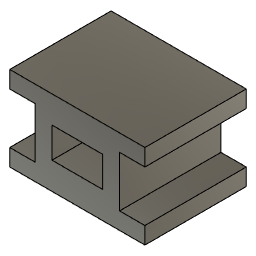
Part 8 (Autodesk Fusion 360 design; units mm, degrees)
Autodesk Fusion 360 part; units mm, degrees
sketch "Sketch2" plane through (0, 0, 0) normal (0, 1, 0) x (1, 0, 0)
  line L0 (40, -25) -> (-40, -25)
  line L1 (-40, -25) -> (-40, 25)
  line L2 (-40, 25) -> (40, 25)
  line L3 (40, 25) -> (40, -25)
  line L4 (40, -25) -> (-40, 25) construction
  line L5 (-40, -25) -> (40, 25) construction
  line L6 (15, -9) -> (-15, -9)
  line L7 (-15, -9) -> (-15, 9)
  line L8 (-15, 9) -> (15, 9)
  line L9 (15, 9) -> (15, -9)
  line L10 (15, -9) -> (-15, 9) construction
  line L11 (-15, -9) -> (15, 9) construction
  line L12 (40, -15) -> (25, -15)
  line L13 (25, -15) -> (25, 15)
  line L14 (25, 15) -> (40, 15)
  line L15 (40, 15) -> (40, -15)
  line L16 (-40, 15) -> (-25, 15)
  line L17 (-25, 15) -> (-25, -15)
  line L18 (-25, -15) -> (-40, -15)
  line L19 (-40, -15) -> (-40, 15)
  dimension "d13" = 80
  dimension "d14" = 50
  dimension "d15" = 30
  dimension "d16" = 18
  dimension "d17" = 15
  dimension "d18" = 30
  dimension "d19" = 10
  constraint horizontal L0
  constraint perpendicular L0 L1
  constraint parallel L0 L2
  constraint parallel L1 L3
  constraint coincident L4 origin
  constraint coincident L5 origin
  constraint horizontal L6
  constraint perpendicular L6 L7
  constraint parallel L6 L8
  constraint parallel L7 L9
  constraint coincident L10 origin
  constraint coincident L11 origin
  constraint horizontal L12
  constraint vertical L13
  constraint horizontal L14
  constraint vertical L15
  constraint coincident L3 L12.start
  constraint horizontal L16
  constraint vertical L17
  constraint horizontal L18
  constraint vertical L19
  constraint coincident L1 L16.start
  constraint equal L14 L16
  constraint collinear L14 L16
  constraint collinear L12 L18
  measures "d13" distance of L1.end L2.end
  measures "d14" distance of L0.end L1.end
  measures "d15" distance of L7.end L8.end
  measures "d16" distance of L6.end L7.end
  measures "d17" distance of L16.start L16.end
  measures "d18" distance of L12.end L13.end
  measures "d19" distance of L2 L16
extrude "Extrude2" add sketch "Sketch2" along normal blind 60 contours L0 L1 L2 L3 L12 L13 L14 L16 L17 L18
